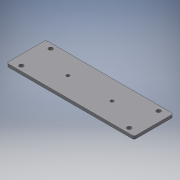
# Autodesk Inventor part: RPlate
Saved by Autodesk Inventor 2018.2 (Build 222227000, 227)
## iProperties
Created: 2018-08-24
Part Number: RPlate
Material: 一般
Document SubType Name: Modeling
Designer: gisen
Density: 1 g/cm^3
Appearance: 既定
Author: gisen
Autodesk Inventor part; units mm, degrees
ref_plane "YZ Plane" through (0, 0, 0) normal (1, 0, 0) x (0, 1, 0)
ref_plane "XZ Plane" through (0, 0, 0) normal (0, 1, 0) x (-1, 0, 0)
ref_plane "XY Plane" through (0, 0, 0) normal (0, 0, 1) x (1, 0, 0)
sketch "スケッチ1" plane through (0, 0, 0) normal (0, 0, 1) x (1, 0, 0)
  line L0 (65, -20) -> (-65, -20)
  line L1 (-65, -20) -> (-65, 20)
  line L2 (-65, 20) -> (65, 20)
  line L3 (65, 20) -> (65, -20)
  line L4 (65, -20) -> (-65, 20) construction
  line L5 (-65, -20) -> (65, 20) construction
  circle A0 centre (-55, 15) radius 2.1
  circle A1 centre (-55, -15) radius 2.1
  circle A2 centre (55, 15) radius 2.1
  circle A3 centre (55, -15) radius 2.1
  circle A4 centre (22.5, 0) radius 1.6
  circle A5 centre (-22.5, 0) radius 1.6
  point P0 (0, 0)
  point P1 (0, 0)
  dimension "d0" = 130
  dimension "d1" = 40
  dimension "d2" = 4.2
  dimension "d3" = 4.2
  dimension "d4" = 4.2
  dimension "d5" = 4.2
  dimension "d6" = 3.2
  dimension "d7" = 3.2
  dimension "d8" = 22.5
  dimension "d9" = 22.5
  dimension "d10" = 10
  dimension "d11" = 10
  dimension "d12" = 5
  dimension "d13" = 5
  dimension "d14" = 10
  dimension "d15" = 5
  dimension "d16" = 10
  dimension "d17" = 5
  constraints: 12 end point, 6 centre point, 3 midpoint, 2 horizontal alignment, 2 parallel, 1 horizontal, 1 perpendicular
  measures "d0" distance of L1.end L2.end
  measures "d1" distance of L0.end L1.end
  measures "d2" diameter of A0
  measures "d3" diameter of A1
  measures "d4" diameter of A2
  measures "d5" diameter of A3
  measures "d6" diameter of A4
  measures "d7" diameter of A5
  measures "d8" distance of A5.centre point (0, 0)
  measures "d9" distance of point (0, 0) A4.centre
  measures "d10" distance from line of L1 A0.centre
  measures "d11" distance from line of L1 A1.centre
  measures "d12" distance from line of L0 A1.centre
  measures "d13" distance from line of L2 A0.centre
  measures "d14" distance from line of L3 A2.centre
  measures "d15" distance from line of L2 A2.centre
  measures "d16" distance from line of L3 A3.centre
  measures "d17" distance from line of L0 A3.centre
extrude "押し出し1" add sketch "スケッチ1" along normal blind 3
fillet "フィレット1" radius 2 4 edges at (65, 20, 1.5) (65, -20, 1.5) (-65, 20, 1.5) (-65, -20, 1.5)
